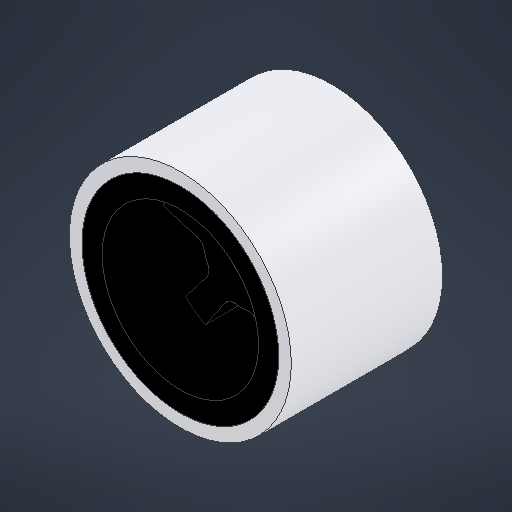
# Autodesk Inventor part: BANH_44
Saved by Autodesk Inventor 2026.1 (Build 301233000, 233)
## iProperties
Created: 2025-09-08
Part Number: BANH_44
Material: Generic
Document SubType Name: Modeling
Designer: ASUS
Density: 1 g/cm^3
Appearance: Default
Author: ASUS
Autodesk Inventor part; units mm, degrees
ref_plane "YZ Plane" through (0, 0, 0) normal (1, 0, 0) x (0, 1, 0)
ref_plane "XZ Plane" through (0, 0, 0) normal (0, 1, 0) x (-1, 0, 0)
sketch "Sketch1" plane through (0, 0, 0) normal (0, 0, 1) x (1, 0, 0)
  circle A0 centre (0, 0) radius 19.5
  circle A1 centre (0, 0) radius 15.5
  dimension "d0" = 39
  dimension "d3" = 31
  constraints: 2 centre point, 2 coincident
  measures "d0" diameter of A0
  measures "d3" diameter of A1
extrude "Extrusion1" add sketch "Sketch1" along normal blind 30
sketch "Sketch2" plane through (0, 0, 30) normal (0, 0, 1) x (1, 0, 0)
  circle A0 centre (0, 0) radius 22
  circle A1 centre (0, 0) radius 19.5
  dimension "d4" = 44
  dimension "d5" = 39
  constraints: 2 centre point, 2 coincident
  measures "d4" diameter of A0
  measures "d5" diameter of A1
extrude "Extrusion2" add sketch "Sketch2" against normal blind 30 separate body
ref_plane "Work Plane1" through (0, 0, 18) normal (0, 0, 1) x (1, 0, 0)
sketch "Sketch3" plane through (0, 0, 18) normal (0, 0, 1) x (1, 0, 0)
  line L0 (2.2444, 8.3814) -> (2.4396, 15.3068)
  circle A0 centre (0, 0) radius 15.5 projected
  line L1 (3.1952, 6.6218) -> (7.2273, 4.1399)
  arc A1 (2.2444, 8.3814) -> (3.1952, 6.6218) centre (4.2436, 8.325) ccw
  line L2 (0, 0) -> (0, 15.5)
  line L3 (-2.2444, 8.3814) -> (-2.4396, 15.3068)
  line L4 (-3.1952, 6.6218) -> (-7.2273, 4.1399)
  arc A2 (-3.1952, 6.6218) -> (-2.2444, 8.3814) centre (-4.2436, 8.325) ccw
  line L5 (-7.2776, 4.7245) -> (-13.8037, 7.0503)
  line L6 (-5.3103, 5.0851) -> (-1.7039, 8.1528)
  arc A3 (-7.2776, 4.7245) -> (-5.3103, 5.0851) centre (-6.6062, 6.6085) ccw
  line L7 (0, 0) -> (-14.7414, 4.7898)
  line L8 (-8.6647, 0.4554) -> (-15.3115, 2.4098)
  line L9 (-7.2851, -0.9926) -> (-6.1706, -5.5943)
  arc A4 (-7.2851, -0.9926) -> (-8.6647, 0.4554) centre (-9.2289, -1.4634) ccw
  line L10 (-6.7422, -5.4614) -> (-10.9708, -10.9495)
  line L11 (-6.4772, -3.4791) -> (-8.2803, 0.8989)
  arc A5 (-6.7422, -5.4614) -> (-6.4772, -3.4791) centre (-8.3265, -4.2407) ccw
  line L12 (0, 0) -> (-9.1107, -12.5398)
  line L13 (-3.1107, -8.0999) -> (-7.0234, -13.8174)
  line L14 (-1.3072, -7.2353) -> (3.4136, -7.5973)
  arc A6 (-1.3072, -7.2353) -> (-3.1107, -8.0999) centre (-1.4602, -9.2294) ccw
  line L15 (3.1107, -8.0999) -> (7.0234, -13.8174)
  line L16 (1.3072, -7.2353) -> (-3.4136, -7.5973)
  arc A7 (3.1107, -8.0999) -> (1.3072, -7.2353) centre (1.4602, -9.2294) ccw
  line L17 (0, 0) -> (9.1107, -12.5398)
  line L18 (6.7422, -5.4614) -> (10.9708, -10.9495)
  line L19 (6.4772, -3.4791) -> (8.2803, 0.8989)
  arc A8 (6.4772, -3.4791) -> (6.7422, -5.4614) centre (8.3265, -4.2407) ccw
  line L20 (8.6647, 0.4554) -> (15.3115, 2.4098)
  line L21 (7.2851, -0.9926) -> (6.1706, -5.5943)
  arc A9 (8.6647, 0.4554) -> (7.2851, -0.9926) centre (9.2289, -1.4634) ccw
  line L22 (0, 0) -> (14.7414, 4.7898)
  line L23 (7.2776, 4.7245) -> (13.8037, 7.0503)
  line L24 (5.3103, 5.0851) -> (1.7039, 8.1528)
  arc A10 (5.3103, 5.0851) -> (7.2776, 4.7245) centre (6.6062, 6.6085) ccw
  point P0 (2.0082, 0)
  point P1 (0.6206, 1.9099)
  point P2 (-1.6246, 1.1804)
  point P3 (-1.6246, -1.1804)
  point P4 (0.6206, -1.9099)
  point P5 (-6.9765, -2.2668)
  point P6 (0, -7.3355)
  point P7 (6.9765, -2.2668)
  point P8 (4.3117, 5.9345)
  point P9 (-4.3117, 5.9345)
  dimension "d13" = 60
  dimension "d15" = 15.3068
  dimension "d17" = 2
  dimension "d20" = 360
  constraints: 50 end point, 22 point on circle, 10 centre point, 5 point on line, 5 symmetric about line, 2 tangent, 1 vertical, 102 other
  measures "d13" angle of L1 L0
  measures "d15" vertical distance of point (2.008, 0) L0.end
  measures "d17" radius of A1
extrude "Extrusion3" add sketch "Sketch3" against normal blind 7 separate body contours A1 L1 L24 A10 L23 A0 L22 L2 L0 | L2 L7 A0 L5 A3 L6 L4 A2 L3 | A0 L20 A9 L21 L19 A8 L18 L17 L22 | L12 A0 L10 A5 L11 L9 A4 L8 L7 | L17 A0 L15 A7 L16 L14 A6 L13 L12
sketch "Sketch4" plane through (0, 0, 11) normal (0, 0, -1) x (-1, 0, 0)
  line L0 (5.993, 2.9012) -> (6.0069, -2.8723)
  line L1 (5.509, -3.7395) -> (0.516, -6.6383)
  line L2 (-0.484, -6.6407) -> (-5.491, -3.766)
  line L3 (-5.993, -2.9012) -> (-6.0069, 2.8723)
  line L4 (-5.509, 3.7395) -> (-0.516, 6.6383)
  line L5 (0.484, 6.6407) -> (5.491, 3.766)
  arc A0 (0.484, 6.6407) -> (-0.516, 6.6383) centre (-0.0139, 5.7735) ccw
  arc A1 (5.993, 2.9012) -> (5.491, 3.766) centre (4.993, 2.8988) ccw
  arc A2 (-5.509, 3.7395) -> (-6.0069, 2.8723) centre (-5.0069, 2.8747) ccw
  arc A3 (-5.993, -2.9012) -> (-5.491, -3.766) centre (-4.993, -2.8988) ccw
  arc A4 (5.509, -3.7395) -> (6.0069, -2.8723) centre (5.0069, -2.8747) ccw
  arc A5 (-0.484, -6.6407) -> (0.516, -6.6383) centre (0.0139, -5.7735) ccw
  point P0 (0, 0)
  point P1 (5.9916, 3.4785)
  point P2 (6.0083, -3.4496)
  point P3 (0.0167, -6.9282)
  point P4 (-5.9916, -3.4785)
  point P5 (-6.0083, 3.4496)
  point P6 (-0.0167, 6.9282)
  dimension "d25" = 12
  dimension "d27" = 1
  dimension "d28" = 1
  constraints: 12 end point, 12 point on circle, 12 point on line, 12 tangent, 6 centre point, 4 equal radius, 13 other
  measures "d25" distance between parallel lines of L0 L3
  measures "d27" radius of A0
  measures "d28" radius of A1
extrude "Extrusion4" cut sketch "Sketch4" against normal blind 4.5 bodies 3
sketch "Sketch5" plane through (0, 0, 18) normal (0, 0, 1) x (1, 0, 0)
  point P0 (0, 0)
  point P1 (0, 0)
  constraints: 1 coincident
hole "Hole1" at (0, 0, 18) direction (0, 0, -1) diameter 3.242 depth 11.8 tip angle 118 bodies 3 thread size "M4x0.7" class "6H" standard "ISO Metric profile"
body "Solid1"
body "Solid2"
body "Solid3"
